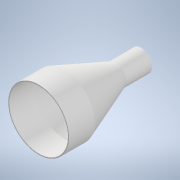
# Autodesk Inventor part: 4.5 to 1.5 inch reducer
Saved by Autodesk Inventor 2021 (Build 250183000, 183)
## iProperties
Created: 2022-05-23
Part Number: 4.5 to 1.5 inch reducer
Material: Generic
Document SubType Name: Modeling
Designer: techv
Density: 1 g/cm^3
Appearance: Default
Author: techv
Autodesk Inventor part; units mm, degrees
ref_plane "YZ Plane" through (0, 0, 0) normal (1, 0, 0) x (0, 1, 0)
ref_plane "XZ Plane" through (0, 0, 0) normal (0, 1, 0) x (-1, 0, 0)
ref_plane "XY Plane" through (0, 0, 0) normal (0, 0, 1) x (1, 0, 0)
sketch "Sketch1" plane through (0, 0, 0) normal (1, 0, 0) x (0, 1, 0)
  line L0 (0, 0) -> (19.05, 0)
  line L1 (19.05, 0) -> (57.15, 100)
  line L2 (57.15, 100) -> (0, 100)
  line L3 (0, 100) -> (0, 0)
  line L4 (0, 0) -> (21.05, 0)
  line L5 (0, 100) -> (59.15, 100)
  line L6 (59.15, 100) -> (21.05, 0)
  line L7 (19.05, 0) -> (19.05, -50)
  line L8 (21.05, 0) -> (21.05, -50)
  line L9 (21.05, -50) -> (19.05, -50)
  line L10 (59.15, 100) -> (59.15, 150)
  line L11 (59.15, 150) -> (57.15, 150)
  line L12 (57.15, 150) -> (57.15, 100)
  dimension "d0" = 19.05
  dimension "d1" = 100
  dimension "d2" = 57.15
  dimension "d3" = 21.05
  dimension "d4" = 59.15
  dimension "d5" = 50
  dimension "d6" = 50
  constraints: 26 end point, 3 perpendicular, 3 vertical, 2 horizontal, 2 parallel, 1 point on line
  measures "d0" distance of L0.start L0.end
  measures "d1" distance between parallel lines of L0 L2
  measures "d2" distance of L1.end L2.end
  measures "d3" distance of L0.start L4.end
  measures "d4" distance of L2.end L5.end
  measures "d5" distance of L0.end L7.end
  measures "d6" distance of L5.end L10.end
revolve "Revolution1" add sketch "Sketch1" angle 360 about axis through (0, 0, 100) along (0, 0, -1) contours L1 L5 L6 L4 | L4 L8 L9 L7 | L12 L11 L10 L5
body "Solid1"
